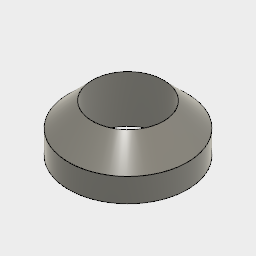
Cuff link v1 (Autodesk Fusion 360 design; units mm, degrees)
Autodesk Fusion 360 part; units mm, degrees
sketch "Sketch1" plane through (0, 0, 0) normal (0, 1, 0) x (1, 0, 0)
  circle A0 centre (0, 0) radius 2.5
  dimension "d1" = 5
  constraint coincident A0.centre origin
  measures "d1" diameter of A0
extrude "Extrude1" add sketch "Sketch1" along normal blind 2
hole "Hole1" at (0, 2, 0) direction (0, -1, 0) diameter 3 end through all
chamfer "Chamfer1" distance 1 angle 45 1 edges at (-2.3308, 2, 0.904)
